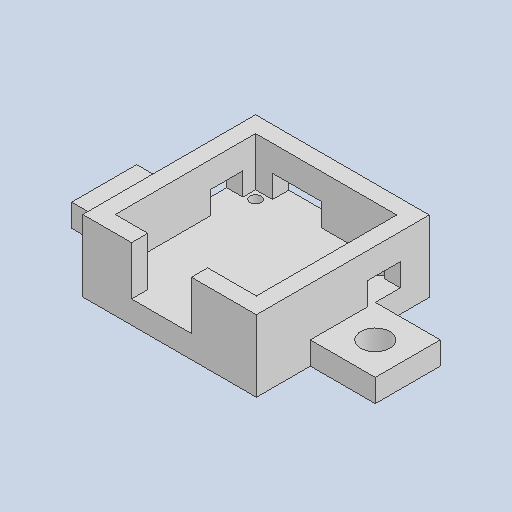
# Autodesk Inventor part: ZED-F9P-02B-case
Saved by Autodesk Inventor 2025.2 (Build 292293000, 293)
## iProperties
Created: 2025-05-12
Part Number: ZED-F9P-02B-case
Material: 일반
Document SubType Name: Modeling
Designer: jbhma
Density: 1 g/cm^3
Appearance: 기본값
Author: jbhma
Autodesk Inventor part; units mm, degrees
ref_plane "YZ Plane" through (0, 0, 0) normal (1, 0, 0) x (0, 1, 0)
ref_plane "XZ Plane" through (0, 0, 0) normal (0, 1, 0) x (-1, 0, 0)
ref_plane "XY Plane" through (0, 0, 0) normal (0, 0, 1) x (1, 0, 0)
sketch "스케치1" plane through (0, 0, 0) normal (0, 1, 0) x (-1, 0, 0)
  line L0 (53.434, 26.59) -> (0, 26.59)
  line L1 (0, 26.59) -> (0, -26.59)
  line L2 (0, -26.59) -> (53.434, -26.59)
  line L3 (53.434, -26.59) -> (53.434, 26.59)
  point P0 (0, 0)
  point P1 (0, 0)
  dimension "d0" = 53.434
  dimension "d1" = 53.18
  constraints: 8 end point, 2 parallel, 1 coincident, 1 horizontal, 1 midpoint, 1 perpendicular
  measures "d0" distance of L2.end L1.end
  measures "d1" distance of L1.end L0.end
extrude "돌출1" add sketch "스케치1" along normal blind 5
sketch "스케치2" plane through (0, 5, 0) normal (0, 1, 0) x (1, 0, 0)
  line L0 (0, -26.59) -> (0, 26.59) projected
  line L1 (0, 26.59) -> (-53.434, 26.59) projected
  line L2 (-53.434, 26.59) -> (-53.434, -26.59) projected
  line L3 (-53.434, -26.59) -> (0, -26.59) projected
  line L4 (-5, -21.59) -> (-48.434, -21.59)
  line L5 (-48.434, -21.59) -> (-48.434, 21.59)
  line L6 (-48.434, 21.59) -> (-5, 21.59)
  line L7 (-5, 21.59) -> (-5, -21.59)
  point P0 (0, 0)
  dimension "d4" = 43.18
  dimension "d5" = 43.434
  dimension "d6" = 5
  dimension "d7" = 5
  constraints: 8 end point, 2 parallel, 1 horizontal, 1 perpendicular
  measures "d4" distance of L4.end L5.end
  measures "d5" distance of L4.start L4.end
  measures "d6" distance between parallel lines of L5 L2
  measures "d7" distance between parallel lines of L3 L4
extrude "돌출2" add sketch "스케치2" along normal blind 15
sketch "스케치3" plane through (-5, 5, 21.59) normal (0, 0, -1) x (-1, 0, 0)
  line L0 (43.434, 0) -> (0, 0) projected
  line L1 (43.434, 0) -> (43.434, 15) projected
  line L2 (0, 15) -> (43.434, 15) projected
  line L3 (0, 0) -> (0, 15) projected
  line L4 (15, 15) -> (33.434, 15)
  line L5 (33.434, 15) -> (33.434, 0)
  line L6 (33.434, 0) -> (15, 0)
  line L7 (15, 0) -> (15, 15)
  point P0 (-5, -5)
  point P1 (15, 0)
  dimension "d10" = 10
  dimension "d11" = 15
  constraints: 8 end point, 2 parallel, 2 point on line, 1 horizontal, 1 perpendicular
  measures "d10" distance between parallel lines of L1 L5
  measures "d11" distance between parallel lines of L7 L3
extrude "돌출3" cut sketch "스케치3" against normal blind 5 contours L0 L7 L2 L5
sketch "스케치4" plane through (-48.434, 5, -21.59) normal (0, 0, 1) x (1, 0, 0)
  line L0 (43.434, 0) -> (0, 0) projected
  line L1 (43.434, 0) -> (43.434, 15) projected
  line L2 (0, 15) -> (43.434, 15) projected
  line L3 (0, 0) -> (0, 15) projected
  line L4 (5.2, 0) -> (20.2, 0)
  line L5 (20.2, 0) -> (20.2, 7)
  line L6 (20.2, 7) -> (5.2, 7)
  line L7 (5.2, 7) -> (5.2, 0)
  point P0 (48.434, -5)
  point P1 (12.7, 0)
  point P2 (20.2, 0)
  dimension "d14" = 12.7
  dimension "d15" = 15
  dimension "d16" = 7
  constraints: 8 end point, 2 parallel, 1 horizontal, 1 midpoint, 1 perpendicular, 1 point on line
  measures "d14" distance from line of L3 point (12.7, 0)
  measures "d15" distance of L5.end L6.end
  measures "d16" distance of L4.end L5.end
extrude "돌출4" cut sketch "스케치4" against normal blind 5 contours L0 L7 L6 L5
sketch "스케치5" plane through (-48.434, 5, 21.59) normal (1, 0, 0) x (0, 0, -1)
  line L0 (43.18, 0) -> (0, 0) projected
  line L1 (43.18, 0) -> (43.18, 15) projected
  line L2 (0, 15) -> (43.18, 15) projected
  line L3 (0, 0) -> (0, 15) projected
  line L4 (29.29, 7) -> (39.29, 7)
  line L5 (39.29, 7) -> (39.29, 0)
  line L6 (39.29, 0) -> (29.29, 0)
  line L7 (29.29, 0) -> (29.29, 7)
  point P0 (21.59, -5)
  point P1 (34.29, 0)
  point P2 (29.29, 0)
  dimension "d19" = 8.89
  dimension "d20" = 10
  dimension "d21" = 7
  constraints: 8 end point, 2 parallel, 1 horizontal, 1 midpoint, 1 perpendicular, 1 point on line
  measures "d19" distance from line of L1 point (34.29, 0)
  measures "d20" distance of L4.start L4.end
  measures "d21" distance of L6.end L4.start
extrude "돌출5" cut sketch "스케치5" along normal mid plane 100 contours L0 L7 L4 L5
sketch "스케치6" plane through (0, 5, 0) normal (0, 1, 0) x (1, 0, 0)
  line L0 (-5, 17.7) -> (-5, 21.59) projected
  line L1 (-5, 21.59) -> (-28.234, 21.59) projected
  line L2 (-28.234, 21.59) -> (-28.234, 26.59) projected
  line L3 (-43.234, 26.59) -> (-28.234, 26.59) projected
  line L4 (-43.234, 21.59) -> (-43.234, 26.59) projected
  line L5 (-43.234, 21.59) -> (-48.434, 21.59) projected
  line L6 (-48.434, 21.59) -> (-48.434, 17.7) projected
  line L7 (-53.434, 17.7) -> (-48.434, 17.7) projected
  line L8 (-53.434, 7.7) -> (-53.434, 17.7) projected
  line L9 (-53.434, 7.7) -> (-48.434, 7.7) projected
  line L10 (-48.434, 7.7) -> (-48.434, -21.59) projected
  line L11 (-48.434, -21.59) -> (-38.434, -21.59) projected
  line L12 (-38.434, -21.59) -> (-38.434, -26.59) projected
  line L13 (-20, -26.59) -> (-38.434, -26.59) projected
  line L14 (-20, -21.59) -> (-20, -26.59) projected
  line L15 (-20, -21.59) -> (-5, -21.59) projected
  line L16 (-5, -21.59) -> (-5, 7.7) projected
  line L17 (-5, 7.7) -> (0, 7.7) projected
  line L18 (0, 17.7) -> (0, 7.7) projected
  line L19 (-5, 17.7) -> (0, 17.7) projected
  circle A0 centre (-45.894, 19.05) radius 1.75
  circle A1 centre (-45.894, -19.05) radius 1.75
  circle A2 centre (-7.54, 19.05) radius 1.75
  circle A3 centre (-7.54, -19.05) radius 1.75
  point P0 (0, 0)
  dimension "d24" = 3.5
  dimension "d25" = 3.5
  dimension "d26" = 3.5
  dimension "d27" = 3.5
  dimension "d28" = 2.54
  dimension "d29" = 2.54
  dimension "d30" = 2.54
  dimension "d31" = 2.54
  dimension "d32" = 2.54
  dimension "d33" = 2.54
  dimension "d34" = 2.54
  dimension "d35" = 2.54
  constraints: 4 centre point
  measures "d24" diameter of A0
  measures "d25" diameter of A1
  measures "d26" diameter of A2
  measures "d27" diameter of A3
  measures "d28" distance from line of A0.centre L5
  measures "d29" distance from line of L6 A0.centre
  measures "d30" distance from line of L10 A1.centre
  measures "d31" distance from line of L11 A1.centre
  measures "d32" distance from line of L15 A3.centre
  measures "d33" distance from line of L16 A3.centre
  measures "d34" distance from line of L1 A2.centre
  measures "d35" distance from line of L0 A2.centre
extrude "돌출6" cut sketch "스케치6" against normal blind 5 contours A0 | A1 | A2 | A3
sketch "스케치7" plane through (0, 0, 26.59) normal (1, 0, 0) x (0, 0, -1)
  line L0 (34.29, 12) -> (44.29, 12) projected
  line L1 (44.29, 12) -> (44.29, 5) projected
  line L2 (44.29, 5) -> (34.29, 5) projected
  line L3 (34.29, 5) -> (34.29, 12) projected
  line L4 (0, 0) -> (53.18, 0) projected
  line L5 (53.18, 0) -> (53.18, 20) projected
  line L6 (0, 20) -> (53.18, 20) projected
  line L7 (0, 0) -> (0, 20) projected
  line L8 (16.59, 0) -> (36.59, 0)
  line L9 (36.59, 0) -> (36.59, 5)
  line L10 (36.59, 5) -> (16.59, 5)
  line L11 (16.59, 5) -> (16.59, 0)
  point P0 (26.59, 0)
  point P1 (26.59, 0)
  dimension "d38" = 20
  dimension "d39" = 5
  constraints: 8 end point, 2 midpoint, 2 parallel, 1 horizontal, 1 perpendicular, 1 point on line
  measures "d38" distance of L10.end L9.end
  measures "d39" distance of L9.end L8.end
extrude "돌출7" add sketch "스케치7" along normal blind 20 contours L2 L9 L4 L11 L10
sketch "스케치8" plane through (-53.434, 0, -26.59) normal (-1, 0, 0) x (0, 0, 1)
  line L0 (8.89, 12) -> (18.89, 12) projected
  line L1 (18.89, 12) -> (18.89, 5) projected
  line L2 (18.89, 5) -> (8.89, 5) projected
  line L3 (8.89, 5) -> (8.89, 12) projected
  line L4 (0, 0) -> (53.18, 0) projected
  line L5 (53.18, 0) -> (53.18, 20) projected
  line L6 (0, 20) -> (53.18, 20) projected
  line L7 (0, 0) -> (0, 20) projected
  line L8 (16.59, 0) -> (36.59, 0)
  line L9 (36.59, 0) -> (36.59, 5)
  line L10 (36.59, 5) -> (16.59, 5)
  line L11 (16.59, 5) -> (16.59, 0)
  point P0 (26.59, 0)
  point P1 (26.59, 0)
  dimension "d42" = 20
  dimension "d43" = 5
  constraints: 8 end point, 2 midpoint, 2 parallel, 1 horizontal, 1 perpendicular, 1 point on line
  measures "d42" distance of L10.end L9.end
  measures "d43" distance of L9.end L8.end
extrude "돌출8" add sketch "스케치8" along normal blind 20 contours L10 L9 L4 L11 L2
sketch "스케치9" plane through (0, 5, 0) normal (0, 1, 0) x (1, 0, 0)
  circle A0 centre (-45.894, -19.05) radius 1.75 projected
  circle A1 centre (-7.54, 19.05) radius 1.75 projected
  circle A2 centre (-7.54, -19.05) radius 1.75 projected
  circle A3 centre (-45.894, 19.05) radius 1.75 projected
  line L0 (-5, 17.7) -> (-5, 21.59) projected
  line L1 (-5, 21.59) -> (-28.234, 21.59) projected
  line L2 (-28.234, 21.59) -> (-28.234, 26.59) projected
  line L3 (-43.234, 26.59) -> (-28.234, 26.59) projected
  line L4 (-43.234, 21.59) -> (-43.234, 26.59) projected
  line L5 (-43.234, 21.59) -> (-48.434, 21.59) projected
  line L6 (-48.434, 21.59) -> (-48.434, 17.7) projected
  line L7 (-53.434, 17.7) -> (-48.434, 17.7) projected
  line L8 (-53.434, 10) -> (-53.434, 17.7) projected
  line L9 (-53.434, 10) -> (-73.434, 10) projected
  line L10 (-73.434, -10) -> (-73.434, 10) projected
  line L11 (-53.434, -10) -> (-73.434, -10) projected
  line L12 (-53.434, 7.7) -> (-53.434, -10) projected
  line L13 (-53.434, 7.7) -> (-48.434, 7.7) projected
  line L14 (-48.434, 7.7) -> (-48.434, -21.59) projected
  line L15 (-48.434, -21.59) -> (-38.434, -21.59) projected
  line L16 (-38.434, -21.59) -> (-38.434, -26.59) projected
  line L17 (-20, -26.59) -> (-38.434, -26.59) projected
  line L18 (-20, -21.59) -> (-20, -26.59) projected
  line L19 (-20, -21.59) -> (-5, -21.59) projected
  line L20 (-5, -21.59) -> (-5, 7.7) projected
  line L21 (-5, 7.7) -> (0, 7.7) projected
  line L22 (0, -10) -> (0, 7.7) projected
  line L23 (0, -10) -> (20, -10) projected
  line L24 (20, 10) -> (20, -10) projected
  line L25 (0, 10) -> (20, 10) projected
  line L26 (0, 17.7) -> (0, 10) projected
  line L27 (-5, 17.7) -> (0, 17.7) projected
  circle A4 centre (10, 0) radius 4.5
  circle A5 centre (-63.434, 0) radius 4.5
  point P0 (0, 0)
  dimension "d46" = 9
  dimension "d47" = 9
  dimension "d48" = 10
  dimension "d49" = 10
  dimension "d50" = 10
  dimension "d51" = 10
  constraints: 2 centre point
  measures "d46" diameter of A4
  measures "d47" diameter of A5
  measures "d48" distance from line of L10 A5.centre
  measures "d49" distance from line of L9 A5.centre
  measures "d50" distance from line of L24 A4.centre
  measures "d51" distance from line of L23 A4.centre
extrude "돌출9" cut sketch "스케치9" against normal blind 5 contours A4 | A5
sketch "스케치10" plane through (0, 0, 0) normal (0, -1, 0) x (1, 0, 0)
  circle A0 centre (-63.434, 0) radius 4.5 projected
  circle A1 centre (10, 0) radius 4.5 projected
  circle A2 centre (-45.894, 19.05) radius 1.75 projected
  circle A3 centre (-7.54, -19.05) radius 1.75 projected
  circle A4 centre (-7.54, 19.05) radius 1.75 projected
  circle A5 centre (-45.894, -19.05) radius 1.75 projected
  line L0 (0, 26.59) -> (0, 10) projected
  line L1 (-53.434, 26.59) -> (0, 26.59) projected
  line L2 (-53.434, 10) -> (-53.434, 26.59) projected
  line L3 (-53.434, 10) -> (-73.434, 10) projected
  line L4 (-73.434, -10) -> (-73.434, 10) projected
  line L5 (-53.434, -10) -> (-73.434, -10) projected
  line L6 (-53.434, -26.59) -> (-53.434, -10) projected
  line L7 (0, -26.59) -> (-53.434, -26.59) projected
  line L8 (0, -10) -> (0, -26.59) projected
  line L9 (0, -10) -> (20, -10) projected
  line L10 (20, 10) -> (20, -10) projected
  line L11 (0, 10) -> (20, 10) projected
  line L12 (-53.434, 26.59) -> (0, 26.59)
  line L13 (0, 26.59) -> (0, -26.59)
  line L14 (0, -26.59) -> (-53.434, -26.59)
  line L15 (-53.434, -26.59) -> (-53.434, 26.59)
  line L16 (0, 10) -> (20, 10)
  line L17 (20, 10) -> (20, -10)
  line L18 (20, -10) -> (0, -10)
  line L19 (0, -10) -> (0, 10)
  line L20 (-73.434, 10) -> (-53.434, 10)
  line L21 (-53.434, 10) -> (-53.434, -10)
  line L22 (-53.434, -10) -> (-73.434, -10)
  line L23 (-73.434, -10) -> (-73.434, 10)
  point P0 (0, 0)
  constraints: 24 end point, 6 parallel, 3 horizontal, 3 perpendicular
extrude "돌출10" add sketch "스케치10" along normal blind 2
